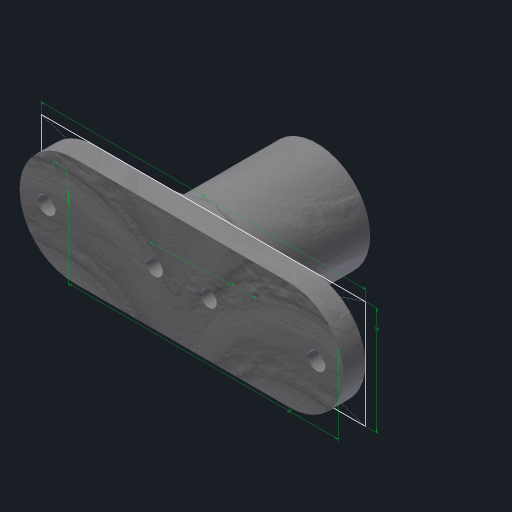
# Autodesk Inventor part: GIRO_1
Saved by Autodesk Inventor 2024.3 (Build 283343000, 343)
## iProperties
Created: 2024-07-12
Part Number: GIRO_1
Material: Steel, Mild, Welded
Document SubType Name: Modeling
Designer: Niler
Density: 7.85 g/cm^3
Appearance: Weld - Steel Mild
Author: Niler
Autodesk Inventor part; units mm, degrees
ref_plane "YZ Plane" through (0, 0, 0) normal (1, 0, 0) x (0, 1, 0)
ref_plane "XZ Plane" through (0, 0, 0) normal (0, 1, 0) x (-1, 0, 0)
ref_plane "XY Plane" through (0, 0, 0) normal (0, 0, 1) x (1, 0, 0)
sketch "Sketch1" plane through (0, 0, 0) normal (0, 0, 1) x (1, 0, 0)
  line L0 (-30, -10) -> (30, -10)
  line L1 (30, -10) -> (30, 10)
  line L2 (30, 10) -> (-30, 10)
  line L3 (-30, 10) -> (-30, -10)
  line L4 (-30, -10) -> (30, 10) construction
  line L5 (30, -10) -> (-30, 10) construction
  circle A0 centre (0, 0) radius 9.9
  circle A1 centre (-25, 0) radius 1.65
  circle A2 centre (25, 0) radius 1.65
  line L6 (-25, 0) -> (25, 0) construction
  point P0 (-30, 0)
  dimension "d0" = 60
  dimension "d1" = 19.8
  dimension "d2" = 20
  dimension "d3" = 50
  dimension "d4" = 3.3
  constraints: 14 end point, 4 midpoint, 3 centre point, 2 horizontal, 2 horizontal alignment, 2 parallel, 1 coincident, 1 equal radius, 1 perpendicular
  measures "d0" distance of L2.end L1.end
  measures "d1" diameter of A0
  measures "d2" distance of L0.end L1.end
  measures "d3" distance of L6.end L6.start
  measures "d4" diameter of A1
extrude "Extrusion1" add sketch "Sketch1" along normal blind 4 contours L3 L2 L1 L0 | A0
extrude "Extrusion2" add sketch "Sketch1" against normal blind 21 contours A0
fillet "Fillet1" radius 2 1 edges at (-9.9, 0, 0)
fillet "Fillet2" radius 10 4 edges at (30, 10, 2) (30, -10, 2) (-30, 10, 2) (-30, -10, 2)
sketch "Sketch2" plane through (0, 0, 0) normal (0, 0, -1) x (-1, 0, 0)
  arc A0 (-20, 10) -> (-20, -10) centre (-20, 0) ccw projected
  line L0 (-6.4506, -10) -> (-20, -10) projected
  arc A1 (-6.4506, 10) -> (-6.4506, -10) centre (0, 0) ccw projected
  line L1 (-20, 10) -> (-6.4506, 10) projected
  circle A2 centre (-25, 0) radius 1.65 projected
  line L2 (25, 0) -> (-25, 0) construction
  line L3 (-23.3257, -2.9) -> (-26.6743, -2.9)
  line L4 (-26.6743, -2.9) -> (-28.3486, 0)
  line L5 (-28.3486, 0) -> (-26.6743, 2.9)
  line L6 (-26.6743, 2.9) -> (-23.3257, 2.9)
  line L7 (-23.3257, 2.9) -> (-21.6514, 0)
  line L8 (-21.6514, 0) -> (-23.3257, -2.9)
  circle A3 centre (25, 0) radius 1.65 projected
  line L9 (23.3257, 2.9) -> (26.6743, 2.9)
  line L10 (26.6743, 2.9) -> (28.3486, 0)
  line L11 (28.3486, 0) -> (26.6743, -2.9)
  line L12 (26.6743, -2.9) -> (23.3257, -2.9)
  line L13 (23.3257, -2.9) -> (21.6514, 0)
  line L14 (21.6514, 0) -> (23.3257, 2.9)
  point P0 (25, 2.9)
  dimension "d11" = 5.8
  dimension "d12" = 5.8
  constraints: 24 end point, 2 coincident, 2 horizontal alignment, 1 midpoint, 26 other
  measures "d11" distance from line of L12 point (25, 2.9)
  measures "d12" distance between parallel lines of L3 L6
extrude "Extrusion3" cut sketch "Sketch2" against normal blind 2 contours L3 L4 L5 L6 L7 L8 | L9 L10 L11 L12 L13 L14
sketch "Sketch3" plane through (0, 0, -21) normal (0, 0, -1) x (-1, 0, 0)
  circle A0 centre (0, 0) radius 9.9 projected
  circle A1 centre (-5, 0) radius 1.5
  line L0 (0, 0) -> (0, 2.4769)
  circle A2 centre (5, 0) radius 1.5
  dimension "d15" = 3
  dimension "d16" = 10
  constraints: 2 centre point, 2 end point, 1 horizontal alignment, 1 symmetric about line, 1 vertical, 1 other
  measures "d15" diameter of A1
  measures "d16" distance of A2.centre A1.centre
extrude "Extrusion4" cut sketch "Sketch3" against normal through all contours A1 | A2
body "Solid1"
